Autodesk Inventor part; units mm, degrees
(part 2 of 2)
sketch "Sketch3" plane through (0, 0, -3.4) normal (0, 0, -1) x (-1, 0, 0)
  line L0 (0, 0) -> (23.6, 0)
  line L1 (23.6, 0) -> (23.6, 65.2958)
  line L2 (23.6, 65.2958) -> (0, 65.2958)
  line L3 (0, 65.2958) -> (0, 0)
  circle A0 centre (13, 35.0012) radius 9.6 construction
  circle A1 centre (8.9947, 46.9477) radius 8 construction
  circle A2 centre (8.9947, 46.9477) radius 8.4
  circle A3 centre (13, 35.0012) radius 10
  circle A4 centre (14.5, 55.2958) radius 5 projected
  circle A5 centre (8.9947, 46.9477) radius 1.25 construction
  arc A6 (9.7521, 54.9117) -> (9.2865, 53.8165) centre (14.0905, 52.4209) ccw construction
  arc A7 (9.2865, 53.8165) -> (8.9266, 53.8223) centre (8.9947, 46.9477) ccw construction
  arc A8 (8.9266, 53.8223) -> (8.4969, 54.9322) centre (4.0798, 52.5838) ccw construction
  arc A9 (8.4969, 54.9322) -> (8.0797, 54.8952) centre (8.9947, 46.9477) ccw construction
  arc A10 (8.0797, 54.8952) -> (7.852, 53.727) centre (12.8412, 53.3608) ccw construction
  arc A11 (7.852, 53.727) -> (7.4988, 53.6579) centre (8.9947, 46.9477) ccw construction
  arc A12 (7.4988, 53.6579) -> (6.8477, 54.6542) centre (3.0154, 51.4388) ccw construction
  arc A13 (6.8477, 54.6542) -> (6.4474, 54.5312) centre (8.9947, 46.9477) ccw construction
  arc A14 (6.4474, 54.5312) -> (6.4675, 53.3413) centre (11.4237, 54.0204) ccw construction
  arc A15 (6.4675, 53.3413) -> (6.1364, 53.2003) centre (8.9947, 46.9477) ccw construction
  arc A16 (6.1364, 53.2003) -> (5.2924, 54.0394) centre (2.2123, 50.0975) ccw construction
  arc A17 (5.2924, 54.0394) -> (4.9263, 53.8359) centre (8.9947, 46.9477) ccw construction
  arc A18 (4.9263, 53.8359) -> (5.1934, 52.6761) centre (9.9002, 54.3708) ccw construction
  arc A19 (5.1934, 52.6761) -> (4.8988, 52.4693) centre (8.9947, 46.9477) ccw construction
  arc A20 (4.8988, 52.4693) -> (3.8988, 53.1147) centre (1.7056, 48.6185) ccw construction
  arc A21 (3.8988, 53.1147) -> (3.5831, 52.8395) centre (8.9947, 46.9477) ccw construction
  arc A22 (3.5831, 52.8395) -> (4.0855, 51.7606) centre (8.337, 54.3968) ccw construction
  arc A23 (4.0855, 51.7606) -> (3.8403, 51.4971) centre (8.9947, 46.9477) ccw construction
  arc A24 (3.8403, 51.4971) -> (2.728, 51.9204) centre (1.5175, 47.0665) ccw construction
  arc A25 (2.728, 51.9204) -> (2.4763, 51.5856) centre (8.9947, 46.9477) ccw construction
  arc A26 (2.4763, 51.5856) -> (3.1921, 50.6348) centre (6.8026, 54.0973) ccw construction
  arc A27 (3.1921, 50.6348) -> (3.0071, 50.326) centre (8.9947, 46.9477) ccw construction
  arc A28 (3.0071, 50.326) -> (1.8311, 50.5088) centre (1.6562, 45.5093) ccw construction
  arc A29 (1.8311, 50.5088) -> (1.6545, 50.129) centre (8.9947, 46.9477) ccw construction
  arc A30 (1.6545, 50.129) -> (2.5523, 49.3477) centre (5.364, 53.4853) ccw construction
  arc A31 (2.5523, 49.3477) -> (2.4355, 49.0073) centre (8.9947, 46.9477) ccw construction
  arc A32 (2.4355, 49.0073) -> (1.2472, 48.9416) centre (2.1156, 44.015) ccw construction
  arc A33 (1.2472, 48.9416) -> (1.1535, 48.5334) centre (8.9947, 46.9477) ccw construction
  arc A34 (1.1535, 48.5334) -> (2.1941, 47.9558) centre (4.0841, 52.5876) ccw construction
  arc A35 (2.1941, 47.9558) -> (2.1506, 47.5985) centre (8.9947, 46.9477) ccw construction
  arc A36 (2.1506, 47.5985) -> (1.002, 47.2872) centre (2.8757, 42.6488) ccw construction
  arc A37 (1.002, 47.2872) -> (0.9951, 46.8684) centre (8.9947, 46.9477) ccw construction
  arc A38 (0.9951, 46.8684) -> (2.1331, 46.5199) centre (3.0188, 51.4434) ccw construction
  arc A39 (2.1331, 46.5199) -> (2.1649, 46.1613) centre (8.9947, 46.9477) ccw construction
  arc A40 (2.1649, 46.1613) -> (1.106, 45.618) centre (3.9032, 41.4705) ccw construction
  arc A41 (1.106, 45.618) -> (1.1864, 45.2069) centre (8.9947, 46.9477) ccw construction
  arc A42 (1.1864, 45.2069) -> (2.372, 45.1026) centre (2.2147, 50.1027) ccw construction
  arc A43 (2.372, 45.1026) -> (2.4776, 44.7585) centre (8.9947, 46.9477) ccw construction
  arc A44 (2.4776, 44.7585) -> (1.5549, 44.0069) centre (5.1532, 40.5316) ccw construction
  arc A45 (1.5549, 44.0069) -> (1.719, 43.6215) centre (8.9947, 46.9477) ccw construction
  arc A46 (1.719, 43.6215) -> (2.9003, 43.7659) centre (1.7069, 48.6241) ccw construction
  arc A47 (2.9003, 43.7659) -> (3.0752, 43.4513) centre (8.9947, 46.9477) ccw construction
  arc A48 (3.0752, 43.4513) -> (2.3289, 42.5243) centre (6.5711, 39.8731) ccw construction
  arc A49 (2.3289, 42.5243) -> (2.5695, 42.1815) centre (8.9947, 46.9477) ccw construction
  arc A50 (2.5695, 42.1815) -> (3.695, 42.5684) centre (1.5176, 47.0722) ccw construction
  arc A51 (3.695, 42.5684) -> (3.9314, 42.297) centre (8.9947, 46.9477) ccw construction
  arc A52 (3.9314, 42.297) -> (3.3942, 41.235) centre (8.095, 39.5238) ccw construction
  arc A53 (3.3942, 41.235) -> (3.7009, 40.9498) centre (8.9947, 46.9477) ccw construction
  arc A54 (3.7009, 40.9498) -> (4.7213, 41.5622) centre (1.6551, 45.5149) ccw construction
  arc A55 (4.7213, 41.5622) -> (5.009, 41.3459) centre (8.9947, 46.9477) ccw construction
  arc A56 (5.009, 41.3459) -> (4.7043, 40.1955) centre (9.6581, 39.499) ccw construction
  arc A57 (4.7043, 40.1955) -> (5.0636, 39.9802) centre (8.9947, 46.9477) ccw construction
  arc A58 (5.0636, 39.9802) -> (5.9344, 40.7914) centre (2.1134, 44.0202) ccw construction
  arc A59 (5.9344, 40.7914) -> (6.2608, 40.6396) centre (8.9947, 46.9477) ccw construction
  arc A60 (6.2608, 40.6396) -> (6.2019, 39.451) centre (11.1923, 39.7997) ccw construction
  arc A61 (6.2019, 39.451) -> (6.5981, 39.3151) centre (8.9947, 46.9477) ccw construction
  arc A62 (6.5981, 39.3151) -> (7.2812, 40.2896) centre (2.8724, 42.6535) ccw construction
  arc A63 (7.2812, 40.2896) -> (7.632, 40.2091) centre (8.9947, 46.9477) ccw construction
  arc A64 (7.632, 40.2091) -> (7.8216, 39.0341) centre (12.6304, 40.4128) ccw construction
  arc A65 (7.8216, 39.0341) -> (8.2374, 38.9836) centre (8.9947, 46.9477) ccw construction
  arc A66 (8.2374, 38.9836) -> (8.703, 40.0789) centre (3.899, 41.4744) ccw construction
  arc A67 (8.703, 40.0789) -> (9.0628, 40.073) centre (8.9947, 46.9477) ccw construction
  arc A68 (9.0628, 40.073) -> (9.4925, 38.9632) centre (13.9097, 41.3115) ccw construction
  arc A69 (9.4925, 38.9632) -> (9.9097, 39.0002) centre (8.9947, 46.9477) ccw construction
  arc A70 (9.9097, 39.0002) -> (10.1374, 40.1683) centre (5.1483, 40.5345) ccw construction
  arc A71 (10.1374, 40.1683) -> (10.4907, 40.2374) centre (8.9947, 46.9477) ccw construction
  arc A72 (10.4907, 40.2374) -> (11.1417, 39.2411) centre (14.9741, 42.4565) ccw construction
  arc A73 (11.1417, 39.2411) -> (11.5421, 39.3641) centre (8.9947, 46.9477) ccw construction
  arc A74 (11.5421, 39.3641) -> (11.522, 40.554) centre (6.5657, 39.875) ccw construction
  arc A75 (11.522, 40.554) -> (11.8531, 40.695) centre (8.9947, 46.9477) ccw construction
  arc A76 (11.8531, 40.695) -> (12.6971, 39.8559) centre (15.7772, 43.7978) ccw construction
  arc A77 (12.6971, 39.8559) -> (13.0632, 40.0594) centre (8.9947, 46.9477) ccw construction
  arc A78 (13.0632, 40.0594) -> (12.7961, 41.2192) centre (8.0893, 39.5245) ccw construction
  arc A79 (12.7961, 41.2192) -> (13.0907, 41.426) centre (8.9947, 46.9477) ccw construction
  arc A80 (13.0907, 41.426) -> (14.0906, 40.7807) centre (16.2839, 45.2768) ccw construction
  arc A81 (14.0906, 40.7807) -> (14.4064, 41.0558) centre (8.9947, 46.9477) ccw construction
  arc A82 (14.4064, 41.0558) -> (13.904, 42.1347) centre (9.6525, 39.4985) ccw construction
  arc A83 (13.904, 42.1347) -> (14.1492, 42.3982) centre (8.9947, 46.9477) ccw construction
  arc A84 (14.1492, 42.3982) -> (15.2615, 41.9749) centre (16.472, 46.8288) ccw construction
  arc A85 (15.2615, 41.9749) -> (15.5131, 42.3097) centre (8.9947, 46.9477) ccw construction
  arc A86 (15.5131, 42.3097) -> (14.7974, 43.2606) centre (11.1869, 39.798) ccw construction
  arc A87 (14.7974, 43.2606) -> (14.9824, 43.5693) centre (8.9947, 46.9477) ccw construction
  arc A88 (14.9824, 43.5693) -> (16.1584, 43.3865) centre (16.3333, 48.386) ccw construction
  arc A89 (16.1584, 43.3865) -> (16.335, 43.7663) centre (8.9947, 46.9477) ccw construction
  arc A90 (16.335, 43.7663) -> (15.4372, 44.5476) centre (12.6255, 40.41) ccw construction
  arc A91 (15.4372, 44.5476) -> (15.554, 44.888) centre (8.9947, 46.9477) ccw construction
  arc A92 (15.554, 44.888) -> (16.7423, 44.9538) centre (15.8739, 49.8803) ccw construction
  arc A93 (16.7423, 44.9538) -> (16.836, 45.362) centre (8.9947, 46.9477) ccw construction
  arc A94 (16.836, 45.362) -> (15.7954, 45.9395) centre (13.9054, 41.3077) ccw construction
  arc A95 (15.7954, 45.9395) -> (15.8389, 46.2968) centre (8.9947, 46.9477) ccw construction
  arc A96 (15.8389, 46.2968) -> (16.9875, 46.6081) centre (15.1138, 51.2465) ccw construction
  arc A97 (16.9875, 46.6081) -> (16.9944, 47.0269) centre (8.9947, 46.9477) ccw construction
  arc A98 (16.9944, 47.0269) -> (15.8564, 47.3755) centre (14.9707, 42.452) ccw construction
  arc A99 (15.8564, 47.3755) -> (15.8246, 47.734) centre (8.9947, 46.9477) ccw construction
  arc A100 (15.8246, 47.734) -> (16.8835, 48.2773) centre (14.0863, 52.4248) ccw construction
  arc A101 (16.8835, 48.2773) -> (16.8031, 48.6884) centre (8.9947, 46.9477) ccw construction
  arc A102 (16.8031, 48.6884) -> (15.6175, 48.7927) centre (15.7748, 43.7927) ccw construction
  arc A103 (15.6175, 48.7927) -> (15.5119, 49.1368) centre (8.9947, 46.9477) ccw construction
  arc A104 (15.5119, 49.1368) -> (16.4346, 49.8884) centre (12.8363, 53.3637) ccw construction
  arc A105 (16.4346, 49.8884) -> (16.2705, 50.2738) centre (8.9947, 46.9477) ccw construction
  arc A106 (16.2705, 50.2738) -> (15.0892, 50.1294) centre (16.2826, 45.2713) ccw construction
  arc A107 (15.0892, 50.1294) -> (14.9143, 50.444) centre (8.9947, 46.9477) ccw construction
  arc A108 (14.9143, 50.444) -> (15.6606, 51.371) centre (11.4184, 54.0222) ccw construction
  arc A109 (15.6606, 51.371) -> (15.42, 51.7138) centre (8.9947, 46.9477) ccw construction
  arc A110 (15.42, 51.7138) -> (14.2945, 51.3269) centre (16.4719, 46.8231) ccw construction
  arc A111 (14.2945, 51.3269) -> (14.058, 51.5983) centre (8.9947, 46.9477) ccw construction
  arc A112 (14.058, 51.5983) -> (14.5953, 52.6603) centre (9.8945, 54.3715) ccw construction
  arc A113 (14.5953, 52.6603) -> (14.2886, 52.9456) centre (8.9947, 46.9477) ccw construction
  arc A114 (14.2886, 52.9456) -> (13.2682, 52.3331) centre (16.3344, 48.3804) ccw construction
  arc A115 (13.2682, 52.3331) -> (12.9805, 52.5494) centre (8.9947, 46.9477) ccw construction
  arc A116 (12.9805, 52.5494) -> (13.2852, 53.6999) centre (8.3314, 54.3963) ccw construction
  arc A117 (13.2852, 53.6999) -> (12.9259, 53.9151) centre (8.9947, 46.9477) ccw construction
  arc A118 (12.9259, 53.9151) -> (12.0551, 53.1039) centre (15.8761, 49.8751) ccw construction
  arc A119 (12.0551, 53.1039) -> (11.7287, 53.2557) centre (8.9947, 46.9477) ccw construction
  arc A120 (11.7287, 53.2557) -> (11.7876, 54.4443) centre (6.7972, 54.0957) ccw construction
  arc A121 (11.7876, 54.4443) -> (11.3914, 54.5802) centre (8.9947, 46.9477) ccw construction
  arc A122 (11.3914, 54.5802) -> (10.7083, 53.6057) centre (15.1171, 51.2419) ccw construction
  arc A123 (10.7083, 53.6057) -> (10.3575, 53.6863) centre (8.9947, 46.9477) ccw construction
  arc A124 (10.3575, 53.6863) -> (10.1679, 54.8612) centre (5.3591, 53.4826) ccw construction
  arc A125 (10.1679, 54.8612) -> (9.7521, 54.9117) centre (8.9947, 46.9477) ccw construction
  arc A126 (6.571, 40.1714) -> (5.2144, 40.6176) centre (4.0302, 34.7325) ccw construction
  arc A127 (5.2144, 40.6176) -> (4.9311, 40.2025) centre (13, 35.0012) ccw construction
  arc A128 (4.9311, 40.2025) -> (5.8414, 39.102) centre (9.9791, 43.4512) ccw construction
  arc A129 (5.8414, 39.102) -> (5.6366, 38.7217) centre (13, 35.0012) ccw construction
  arc A130 (5.6366, 38.7217) -> (4.2168, 38.8762) centre (4.2821, 32.8735) ccw construction
  arc A131 (4.2168, 38.8762) -> (4.026, 38.4112) centre (13, 35.0012) ccw construction
  arc A132 (4.026, 38.4112) -> (5.1452, 37.524) centre (8.2882, 42.6385) ccw construction
  arc A133 (5.1452, 37.524) -> (5.0239, 37.1095) centre (13, 35.0012) ccw construction
  arc A134 (5.0239, 37.1095) -> (3.6031, 36.9654) centre (4.915, 31.1074) ccw construction
  arc A135 (3.6031, 36.9654) -> (3.5132, 36.4709) centre (13, 35.0012) ccw construction
  arc A136 (3.5132, 36.4709) -> (4.7923, 35.8358) centre (6.8033, 41.492) ccw construction
  arc A137 (4.7923, 35.8358) -> (4.7599, 35.4051) centre (13, 35.0012) ccw construction
  arc A138 (4.7599, 35.4051) -> (3.4001, 34.9687) centre (5.9012, 29.5115) ccw construction
  arc A139 (3.4001, 34.9687) -> (3.4149, 34.4663) centre (13, 35.0012) ccw construction
  arc A140 (3.4149, 34.4663) -> (4.7982, 34.1111) centre (5.5892, 40.0618) ccw construction
  arc A141 (4.7982, 34.1111) -> (4.856, 33.6831) centre (13, 35.0012) ccw construction
  arc A142 (4.856, 33.6831) -> (3.6166, 32.9735) centre (7.1977, 28.1556) ccw construction
  arc A143 (3.6166, 32.9735) -> (3.7356, 32.4852) centre (13, 35.0012) ccw construction
  arc A144 (3.7356, 32.4852) -> (5.1625, 32.4253) centre (4.699, 38.4104) ccw construction
  arc A145 (5.1625, 32.4253) -> (5.308, 32.0186) centre (13, 35.0012) ccw construction
  arc A146 (5.308, 32.0186) -> (4.2432, 31.0669) centre (8.7478, 27.0988) ccw construction
  arc A147 (4.2432, 31.0669) -> (4.4611, 30.614) centre (13, 35.0012) ccw construction
  arc A148 (4.4611, 30.614) -> (5.8693, 30.8521) centre (4.1716, 36.61) ccw construction
  arc A149 (5.8693, 30.8521) -> (6.0962, 30.4845) centre (13, 35.0012) ccw construction
  arc A150 (6.0962, 30.4845) -> (5.2526, 29.3322) centre (10.4837, 26.3874) ccw construction
  arc A151 (5.2526, 29.3322) -> (5.5599, 28.9345) centre (13, 35.0012) ccw construction
  arc A152 (5.5599, 28.9345) -> (6.8878, 29.4602) centre (4.03, 34.7394) ccw construction
  arc A153 (6.8878, 29.4602) -> (7.1861, 29.1479) centre (13, 35.0012) ccw construction
  arc A154 (7.1861, 29.1479) -> (6.6005, 27.8453) centre (12.3296, 26.0525) ccw construction
  arc A155 (6.6005, 27.8453) -> (6.9838, 27.5202) centre (13, 35.0012) ccw construction
  arc A156 (6.9838, 27.5202) -> (8.1734, 28.3104) centre (4.2805, 32.8801) ccw construction
  arc A157 (8.1734, 28.3104) -> (8.5302, 28.067) centre (13, 35.0012) ccw construction
  arc A158 (8.5302, 28.067) -> (8.2282, 26.6712) centre (14.2048, 26.1086) ccw construction
  arc A159 (8.2282, 26.6712) -> (8.6707, 26.4328) centre (13, 35.0012) ccw construction
  arc A160 (8.6707, 26.4328) -> (9.6699, 27.4531) centre (4.912, 31.1136) ccw construction
  arc A161 (9.6699, 27.4531) -> (10.0695, 27.2892) centre (13, 35.0012) ccw construction
  arc A162 (10.0695, 27.2892) -> (10.0643, 25.8611) centre (16.0273, 26.5534) ccw construction
  arc A163 (10.0643, 25.8611) -> (10.5467, 25.72) centre (13, 35.0012) ccw construction
  arc A164 (10.5467, 25.72) -> (11.312, 26.9257) centre (5.897, 29.5169) ccw construction
  arc A165 (11.312, 26.9257) -> (11.737, 26.8485) centre (13, 35.0012) ccw construction
  arc A166 (11.737, 26.8485) -> (12.0288, 25.4504) centre (17.7176, 27.3675) ccw construction
  arc A167 (12.0288, 25.4504) -> (12.53, 25.4127) centre (13, 35.0012) ccw construction
  arc A168 (12.53, 25.4127) -> (13.0279, 26.7512) centre (7.1925, 28.16) ccw construction
  arc A169 (13.0279, 26.7512) -> (13.4596, 26.764) centre (13, 35.0012) ccw construction
  arc A170 (13.4596, 26.764) -> (14.0358, 25.4572) centre (19.2016, 28.5151) ccw construction
  arc A171 (14.0358, 25.4572) -> (14.5338, 25.5245) centre (13, 35.0012) ccw construction
  arc A172 (14.5338, 25.5245) -> (14.7426, 26.9373) centre (8.7418, 27.102) ccw construction
  arc A173 (14.7426, 26.9373) -> (15.1622, 27.0396) centre (13, 35.0012) ccw construction
  arc A174 (15.1622, 27.0396) -> (15.9974, 25.8811) centre (20.4146, 29.9462) ccw construction
  arc A175 (15.9974, 25.8811) -> (16.4706, 26.0505) centre (13, 35.0012) ccw construction
  arc A176 (16.4706, 26.0505) -> (16.3811, 27.4758) centre (10.4772, 26.3893) ccw construction
  arc A177 (16.3811, 27.4758) -> (16.7703, 27.6631) centre (13, 35.0012) ccw construction
  arc A178 (16.7703, 27.6631) -> (17.8281, 26.7036) centre (21.3036, 31.5983) ccw construction
  arc A179 (17.8281, 26.7036) -> (18.2557, 26.9677) centre (13, 35.0012) ccw construction
  arc A180 (18.2557, 26.9677) -> (17.8718, 28.3432) centre (12.3228, 26.053) ccw construction
  arc A181 (17.8718, 28.3432) -> (18.2136, 28.6073) centre (13, 35.0012) ccw construction
  arc A182 (18.2136, 28.6073) -> (19.4477, 27.8888) centre (21.8296, 33.3991) ccw construction
  arc A183 (19.4477, 27.8888) -> (19.8111, 28.236) centre (13, 35.0012) ccw construction
  arc A184 (19.8111, 28.236) -> (19.1496, 29.5016) centre (14.198, 26.1077) ccw construction
  arc A185 (19.1496, 29.5016) -> (19.429, 29.831) centre (13, 35.0012) ccw construction
  arc A186 (19.429, 29.831) -> (20.7856, 29.3848) centre (21.9698, 35.2699) ccw construction
  arc A187 (20.7856, 29.3848) -> (21.0689, 29.7999) centre (13, 35.0012) ccw construction
  arc A188 (21.0689, 29.7999) -> (20.1586, 30.9004) centre (16.0209, 26.5512) ccw construction
  arc A189 (20.1586, 30.9004) -> (20.3634, 31.2807) centre (13, 35.0012) ccw construction
  arc A190 (20.3634, 31.2807) -> (21.7832, 31.1262) centre (21.7179, 37.1289) ccw construction
  arc A191 (21.7832, 31.1262) -> (21.974, 31.5912) centre (13, 35.0012) ccw construction
  arc A192 (21.974, 31.5912) -> (20.8548, 32.4784) centre (17.7118, 27.3639) ccw construction
  arc A193 (20.8548, 32.4784) -> (20.9761, 32.8929) centre (13, 35.0012) ccw construction
  arc A194 (20.9761, 32.8929) -> (22.3969, 33.037) centre (21.085, 38.895) ccw construction
  arc A195 (22.3969, 33.037) -> (22.4868, 33.5315) centre (13, 35.0012) ccw construction
  arc A196 (22.4868, 33.5315) -> (21.2077, 34.1666) centre (19.1967, 28.5104) ccw construction
  arc A197 (21.2077, 34.1666) -> (21.2401, 34.5973) centre (13, 35.0012) ccw construction
  arc A198 (21.2401, 34.5973) -> (22.5999, 35.0337) centre (20.0988, 40.4909) ccw construction
  arc A199 (22.5999, 35.0337) -> (22.5851, 35.5361) centre (13, 35.0012) ccw construction
  arc A200 (22.5851, 35.5361) -> (21.2018, 35.8913) centre (20.4108, 29.9406) ccw construction
  arc A201 (21.2018, 35.8913) -> (21.144, 36.3193) centre (13, 35.0012) ccw construction
  arc A202 (21.144, 36.3193) -> (22.3834, 37.0289) centre (18.8023, 41.8468) ccw construction
  arc A203 (22.3834, 37.0289) -> (22.2644, 37.5172) centre (13, 35.0012) ccw construction
  arc A204 (22.2644, 37.5172) -> (20.8375, 37.5771) centre (21.301, 31.592) ccw construction
  arc A205 (20.8375, 37.5771) -> (20.692, 37.9838) centre (13, 35.0012) ccw construction
  arc A206 (20.692, 37.9838) -> (21.7568, 38.9355) centre (17.2522, 42.9036) ccw construction
  arc A207 (21.7568, 38.9355) -> (21.5389, 39.3884) centre (13, 35.0012) ccw construction
  arc A208 (21.5389, 39.3884) -> (20.1307, 39.1503) centre (21.8284, 33.3924) ccw construction
  arc A209 (20.1307, 39.1503) -> (19.9038, 39.5178) centre (13, 35.0012) ccw construction
  arc A210 (19.9038, 39.5178) -> (20.7474, 40.6702) centre (15.5163, 43.615) ccw construction
  arc A211 (20.7474, 40.6702) -> (20.4401, 41.0679) centre (13, 35.0012) ccw construction
  arc A212 (20.4401, 41.0679) -> (19.1122, 40.5422) centre (21.97, 35.263) ccw construction
  arc A213 (19.1122, 40.5422) -> (18.8139, 40.8545) centre (13, 35.0012) ccw construction
  arc A214 (18.8139, 40.8545) -> (19.3995, 42.1571) centre (13.6704, 43.9499) ccw construction
  arc A215 (19.3995, 42.1571) -> (19.0162, 42.4822) centre (13, 35.0012) ccw construction
  arc A216 (19.0162, 42.4822) -> (17.8266, 41.692) centre (21.7195, 37.1223) ccw construction
  arc A217 (17.8266, 41.692) -> (17.4698, 41.9354) centre (13, 35.0012) ccw construction
  arc A218 (17.4698, 41.9354) -> (17.7718, 43.3312) centre (11.7952, 43.8938) ccw construction
  arc A219 (17.7718, 43.3312) -> (17.3293, 43.5696) centre (13, 35.0012) ccw construction
  arc A220 (17.3293, 43.5696) -> (16.3301, 42.5493) centre (21.088, 38.8888) ccw construction
  arc A221 (16.3301, 42.5493) -> (15.9305, 42.7132) centre (13, 35.0012) ccw construction
  arc A222 (15.9305, 42.7132) -> (15.9357, 44.1413) centre (9.9727, 43.4489) ccw construction
  arc A223 (15.9357, 44.1413) -> (15.4533, 44.2824) centre (13, 35.0012) ccw construction
  arc A224 (15.4533, 44.2824) -> (14.688, 43.0767) centre (20.103, 40.4855) ccw construction
  arc A225 (14.688, 43.0767) -> (14.263, 43.1539) centre (13, 35.0012) ccw construction
  arc A226 (14.263, 43.1539) -> (13.9712, 44.5519) centre (8.2824, 42.6349) ccw construction
  arc A227 (13.9712, 44.5519) -> (13.47, 44.5897) centre (13, 35.0012) ccw construction
  arc A228 (13.47, 44.5897) -> (12.9721, 43.2512) centre (18.8075, 41.8424) ccw construction
  arc A229 (12.9721, 43.2512) -> (12.5404, 43.2384) centre (13, 35.0012) ccw construction
  arc A230 (12.5404, 43.2384) -> (11.9642, 44.5452) centre (6.7984, 41.4873) ccw construction
  arc A231 (11.9642, 44.5452) -> (11.4662, 44.4779) centre (13, 35.0012) ccw construction
  arc A232 (11.4662, 44.4779) -> (11.2574, 43.0651) centre (17.2582, 42.9004) ccw construction
  arc A233 (11.2574, 43.0651) -> (10.8378, 42.9628) centre (13, 35.0012) ccw construction
  arc A234 (10.8378, 42.9628) -> (10.0026, 44.1213) centre (5.5854, 40.0562) ccw construction
  arc A235 (10.0026, 44.1213) -> (9.5294, 43.9519) centre (13, 35.0012) ccw construction
  arc A236 (9.5294, 43.9519) -> (9.6189, 42.5266) centre (15.5228, 43.6131) ccw construction
  arc A237 (9.6189, 42.5266) -> (9.2297, 42.3393) centre (13, 35.0012) ccw construction
  arc A238 (9.2297, 42.3393) -> (8.1719, 43.2988) centre (4.6964, 38.4041) ccw construction
  arc A239 (8.1719, 43.2988) -> (7.7443, 43.0347) centre (13, 35.0012) ccw construction
  arc A240 (7.7443, 43.0347) -> (8.1282, 41.6591) centre (13.6772, 43.9494) ccw construction
  arc A241 (8.1282, 41.6591) -> (7.7864, 41.3951) centre (13, 35.0012) ccw construction
  arc A242 (7.7864, 41.3951) -> (6.5523, 42.1136) centre (4.1704, 36.6033) ccw construction
  arc A243 (6.5523, 42.1136) -> (6.1889, 41.7664) centre (13, 35.0012) ccw construction
  arc A244 (6.1889, 41.7664) -> (6.8504, 40.5008) centre (11.802, 43.8947) ccw construction
  arc A245 (6.8504, 40.5008) -> (6.571, 40.1714) centre (13, 35.0012) ccw construction
  point P0 (16.2655, 43.6106)
  point P1 (4.3207, 39.9681)
  point P2 (16.9313, 44.196)
  point P3 (16.846, 48.4834)
  point P4 (16.5028, 50.7145)
  point P5 (9.5001, 55.3324)
  dimension "d21" = 0.4
  dimension "d22" = 0.4
  constraints: 8 end point, 3 centre point, 3 point on circle, 2 coincident, 2 parallel, 1 horizontal, 1 perpendicular, 3 other
  measures "d21" radial gap between concentric circles of A1 A2
extrude "Extrusion7" add sketch "Sketch3" along normal blind 3.7
sketch "Sketch12" plane through (-34.0123, 35.7835, 2.1) normal (0, 0, -1) x (-0.6427876, 0.7660444, 0)
  circle A0 centre (-7.5288, 26.3408) radius 1.25 construction
  arc A1 (-9.9487, 22.908) -> (-8.8528, 23.817) centre (-11.7217, 26.1608) ccw construction
  arc A2 (-8.8528, 23.817) -> (-8.512, 23.6657) centre (-7.5288, 26.3408) ccw construction
  arc A3 (-8.512, 23.6657) -> (-8.4509, 22.2432) centre (-4.8493, 23.1107) ccw construction
  arc A4 (-8.4509, 22.2432) -> (-7.9081, 22.1579) centre (-7.5288, 26.3408) ccw construction
  arc A5 (-7.9081, 22.1579) -> (-7.4135, 23.4931) centre (-11.0699, 24.0884) ccw construction
  arc A6 (-7.4135, 23.4931) -> (-7.0428, 23.5325) centre (-7.5288, 26.3408) ccw construction
  arc A7 (-7.0428, 23.5325) -> (-6.2786, 22.3311) centre (-3.5933, 24.8832) ccw construction
  arc A8 (-6.2786, 22.3311) -> (-5.7659, 22.5286) centre (-7.5288, 26.3408) ccw construction
  arc A9 (-5.7659, 22.5286) -> (-6.0051, 23.9322) centre (-9.4693, 22.6196) ccw construction
  arc A10 (-6.0051, 23.9322) -> (-5.7038, 24.1517) centre (-7.5288, 26.3408) ccw construction
  arc A11 (-5.7038, 24.1517) -> (-4.4412, 23.4934) centre (-3.3917, 27.0462) ccw construction
  arc A12 (-4.4412, 23.4934) -> (-4.096, 23.9208) centre (-7.5288, 26.3408) ccw construction
  arc A13 (-4.096, 23.9208) -> (-5.005, 25.0167) centre (-7.3488, 22.1479) ccw construction
  arc A14 (-5.005, 25.0167) -> (-4.8538, 25.3575) centre (-7.5288, 26.3408) ccw construction
  arc A15 (-4.8538, 25.3575) -> (-3.4312, 25.4187) centre (-4.2987, 29.0202) ccw construction
  arc A16 (-3.4312, 25.4187) -> (-3.3459, 25.9614) centre (-7.5288, 26.3408) ccw construction
  arc A17 (-3.3459, 25.9614) -> (-4.6811, 26.456) centre (-5.2764, 22.7996) ccw construction
  arc A18 (-4.6811, 26.456) -> (-4.7205, 26.8267) centre (-7.5288, 26.3408) ccw construction
  arc A19 (-4.7205, 26.8267) -> (-3.5192, 27.591) centre (-6.0712, 30.2763) ccw construction
  arc A20 (-3.5192, 27.591) -> (-3.7166, 28.1036) centre (-7.5288, 26.3408) ccw construction
  arc A21 (-3.7166, 28.1036) -> (-5.1202, 27.8644) centre (-3.8076, 24.4002) ccw construction
  arc A22 (-5.1202, 27.8644) -> (-5.3397, 28.1657) centre (-7.5288, 26.3408) ccw construction
  arc A23 (-5.3397, 28.1657) -> (-4.6814, 29.4283) centre (-8.2342, 30.4778) ccw construction
  arc A24 (-4.6814, 29.4283) -> (-5.1088, 29.7735) centre (-7.5288, 26.3408) ccw construction
  arc A25 (-5.1088, 29.7735) -> (-6.2047, 28.8645) centre (-3.3359, 26.5207) ccw construction
  arc A26 (-6.2047, 28.8645) -> (-6.5455, 29.0158) centre (-7.5288, 26.3408) ccw construction
  arc A27 (-6.5455, 29.0158) -> (-6.6067, 30.4383) centre (-10.2082, 29.5708) ccw construction
  arc A28 (-6.6067, 30.4383) -> (-7.1494, 30.5236) centre (-7.5288, 26.3408) ccw construction
  arc A29 (-7.1494, 30.5236) -> (-7.644, 29.1884) centre (-3.9876, 28.5931) ccw construction
  arc A30 (-7.644, 29.1884) -> (-8.0147, 29.149) centre (-7.5288, 26.3408) ccw construction
  arc A31 (-8.0147, 29.149) -> (-8.779, 30.3504) centre (-11.4643, 27.7983) ccw construction
  arc A32 (-8.779, 30.3504) -> (-9.2916, 30.1529) centre (-7.5288, 26.3408) ccw construction
  arc A33 (-9.2916, 30.1529) -> (-9.0524, 28.7493) centre (-5.5882, 30.0619) ccw construction
  arc A34 (-9.0524, 28.7493) -> (-9.3537, 28.5298) centre (-7.5288, 26.3408) ccw construction
  arc A35 (-9.3537, 28.5298) -> (-10.6163, 29.1881) centre (-11.6658, 25.6353) ccw construction
  arc A36 (-10.6163, 29.1881) -> (-10.9615, 28.7607) centre (-7.5288, 26.3408) ccw construction
  arc A37 (-10.9615, 28.7607) -> (-10.0525, 27.6648) centre (-7.7088, 30.5336) ccw construction
  arc A38 (-10.0525, 27.6648) -> (-10.2038, 27.324) centre (-7.5288, 26.3408) ccw construction
  arc A39 (-10.2038, 27.324) -> (-11.6263, 27.2628) centre (-10.7588, 23.6613) ccw construction
  arc A40 (-11.6263, 27.2628) -> (-11.7116, 26.7201) centre (-7.5288, 26.3408) ccw construction
  arc A41 (-11.7116, 26.7201) -> (-10.3764, 26.2255) centre (-9.7811, 29.8819) ccw construction
  arc A42 (-10.3764, 26.2255) -> (-10.337, 25.8548) centre (-7.5288, 26.3408) ccw construction
  arc A43 (-10.337, 25.8548) -> (-11.5384, 25.0905) centre (-8.9863, 22.4052) ccw construction
  arc A44 (-11.5384, 25.0905) -> (-11.3409, 24.5779) centre (-7.5288, 26.3408) ccw construction
  arc A45 (-11.3409, 24.5779) -> (-9.9373, 24.8171) centre (-11.2499, 28.2813) ccw construction
  arc A46 (-9.9373, 24.8171) -> (-9.7178, 24.5158) centre (-7.5288, 26.3408) ccw construction
  arc A47 (-9.7178, 24.5158) -> (-10.3761, 23.2532) centre (-6.8233, 22.2037) ccw construction
  arc A48 (-10.3761, 23.2532) -> (-9.9487, 22.908) centre (-7.5288, 26.3408) ccw construction
  circle A49 centre (-7.5288, 26.3408) radius 4.2 construction
  circle A50 centre (-7.5288, 26.3408) radius 4.6
  point P0 (-49.2745, 3.0538)
  dimension "d128" = 0.4
  constraints: 1 centre point, 1 coincident, 3 other
extrude "Extrusion11" add sketch "Sketch12" along normal blind 1.5
ref_plane "Work Plane8" through (-34.0123, -5.0123, 0) normal (0, 0, -1) x (0.6427876, 0.7660444, 0)
sketch "Sketch4" plane through (0, 0, -7.1) normal (0, 0, -1) x (-1, 0, 0)
  line L0 (1.5, 0.5) -> (1.5, 16.5) projected
  line L1 (2.5, 0.5) -> (1.5, 0.5) projected
  line L2 (2.5, 16.5) -> (2.5, 0.5) projected
  line L3 (2.5, 16.5) -> (1.5, 16.5) projected
  line L4 (2.5, 16.5) -> (2.5, 17)
  line L5 (2.5, 17) -> (1, 17)
  line L6 (1, 17) -> (1, 0.5)
  line L7 (23.6, 0) -> (0, 0) projected
  line L8 (1, 0.5) -> (1.5, 0.5)
  dimension "d27" = 0.5
  dimension "d28" = 0.5
  constraints: 8 end point, 2 perpendicular, 1 collinear, 1 vertical
  measures "d27" distance between parallel lines of L5 L3
  measures "d28" distance between parallel lines of L6 L0
extrude "Extrusion8" cut sketch "Sketch4" against normal blind 7.1
sketch "Sketch9" plane through (0, 0, 0.6) normal (0, 0, -1) x (-1, 0, 0)
  arc A0 (9.5001, 55.3324) -> (4.3207, 39.9681) centre (8.9947, 46.9477) ccw projected
  point P0 (0, 0)
  point P1 (16.9313, 44.196)
hole "Hole3" at (-8.9947, 46.9477, 0.6) direction (0, 0, 1) diameter 2.5 depth 1.3
sketch "Sketch5" plane through (0, 0, -7.1) normal (0, 0, -1) x (-1, 0, 0)
  line L0 (1.5, 0.5) -> (1.5, 16.5) projected
  line L1 (2.5, 0.5) -> (1.5, 0.5) projected
  line L2 (2.5, 16.5) -> (2.5, 0.5) projected
  line L3 (2.5, 16.5) -> (1.5, 16.5) projected
  line L4 (2.5, 16.5) -> (2.5, 18)
  line L5 (2.5, 18) -> (0, 18)
  line L6 (0, 0) -> (0, 65.2958) projected
  line L7 (0, 0) -> (0, 18)
  line L8 (0, 0) -> (2.5, 0)
  line L9 (2.5, 0) -> (2.5, 0.5)
  line L10 (1, 17) -> (1, 0)
  line L11 (1, 0) -> (3, 0)
  line L12 (3, 0) -> (3, 17)
  line L13 (3, 17) -> (1, 17)
  line L14 (1.5, 13.4) -> (1.5, 9.9) projected
  line L15 (1.5, 13.4) -> (0, 13.4) projected
  line L16 (0, 9.9) -> (0, 13.4) projected
  line L17 (1.5, 9.9) -> (0, 9.9) projected
  line L18 (1.5, 7.1) -> (1.5, 3.6) projected
  line L19 (1.5, 7.1) -> (0, 7.1) projected
  line L20 (0, 3.6) -> (0, 7.1) projected
  line L21 (1.5, 3.6) -> (0, 3.6) projected
  line L22 (-0.5, 13.9) -> (2, 13.9)
  line L23 (2, 13.9) -> (2, 9.4)
  line L24 (2, 9.4) -> (-0.5, 9.4)
  line L25 (-0.5, 9.4) -> (-0.5, 13.9)
  line L26 (-0.5, 7.6) -> (2, 7.6)
  line L27 (2, 7.6) -> (2, 3.1)
  line L28 (2, 3.1) -> (-0.5, 3.1)
  line L29 (-0.5, 3.1) -> (-0.5, 7.6)
  line L30 (1.5, 0.5) -> (1, 0.5)
  point P0 (0, 13.9)
  point P1 (1, 13.9)
  point P2 (2.5, 17)
  point P3 (0, 7.6)
  point P4 (1, 7.6)
  point P5 (1, 9.4)
  point P6 (0, 9.4)
  point P7 (1, 3.1)
  point P8 (0, 3.1)
  point P9 (0, 3.1)
  point P10 (0, 7.6)
  point P11 (2.5, 0)
  point P12 (1, 0)
  dimension "d31" = 0.5
  dimension "d32" = 1
  dimension "d33" = 0.5
  dimension "d34" = 0.5
  constraints: 36 end point, 3 perpendicular, 3 point on line, 2 collinear, 1 vertical, 9 other
  measures "d31" distance between parallel lines of L0 L10
  measures "d32" distance between parallel lines of L5 L13
  measures "d33" distance between parallel lines of L15 L22
  measures "d34" distance between parallel lines of L19 L26
ref_plane "Work Plane6" through (-2.5, 0.5, -17) normal (0, 0, -1) x (0, 1, 0)
extrude "Extrusion9" add sketch "Sketch5" along normal blind 8 contours L1 L9 L8 L10 L30 | L10 L8 L6 L28 | L13 L10 L22 L6 L5 L4
sketch "Sketch7" plane through (0, 0, -7.1) normal (0, 0, -1) x (-1, 0, 0)
  circle A0 centre (8.3716, 60.4381) radius 1.0564 projected
  circle A1 centre (20.6284, 50.1535) radius 1.0564 projected
  circle A2 centre (14.5, 55.2958) radius 5 projected
  circle A3 centre (14.5, 55.2958) radius 13.85 projected
  circle A4 centre (8.3716, 60.4381) radius 2.25
  circle A5 centre (20.6284, 50.1535) radius 2.25
  point P0 (0, 0)
  dimension "d132" = 4.5
  dimension "d133" = 4.5
  constraints: 2 centre point, 2 coincident
  measures "d132" diameter of A4
  measures "d133" diameter of A5
extrude "Extrusion10" cut sketch "Sketch7" against normal blind 2.7 contours A0 | A1 | A4 | A5
sketch "Sketch8" plane through (-8.3716, 63.2121, -4.4) normal (0, 0, -1) x (-1, 0, 0)
  circle A0 centre (0, -2.774) radius 1.0564 projected
  circle A1 centre (12.2567, -13.0586) radius 1.0564 projected
  circle A2 centre (6.1284, -7.9163) radius 5 projected
  circle A3 centre (6.1284, -7.9163) radius 13.85 projected
  point P0 (-8.3716, -63.2121)
  point P1 (0, 0)
  point P2 (12.2567, -10.2846)
hole "Hole2" at (-20.6284, 50.1535, -4.4) at (-8.3716, 60.4381, -4.4) direction (0, 0, 1) diameter 2.5 depth 8.8 counterbore diameter 4.5 counterbore depth 2.5
sketch "Sketch6" plane through (-23.6, 65.2958, 2.1) normal (0, 1, 0) x (1, 0, 0)
  line L0 (0, 9.2) -> (0, 0) projected
  line L1 (23.6, 0) -> (0, 0) projected
  line L2 (0, 4.6) -> (23.6, 4.6)
  line L3 (0.6, 9.2) -> (20.6, 9.2) projected
  line L4 (17.6, 9.2) -> (17.6, 0)
  circle A0 centre (11.1, 4.6) radius 3.5
  circle A1 centre (3.5, 4.6) radius 3.5
  line L5 (23.6, 9.2) -> (23.6, 0) projected
  line L6 (0, 9.2) -> (23.6, 9.2) projected
  point P0 (23.6, 2.1)
  point P1 (11.8, 4.6)
  point P2 (19.8, 4.6)
  point P3 (19.2793, 9.2)
  point P4 (6.6687, 9.2)
  dimension "d52" = 7
  dimension "d53" = 7
  dimension "d55" = 0
  dimension "d67" = 3
  dimension "d102" = 6
  constraints: 5 point on line, 4 end point, 3 midpoint, 2 centre point, 1 perpendicular
  measures "d52" diameter of A1
  measures "d53" diameter of A0
  measures "d55" distance edge to line of A1 L0
  measures "d67" distance edge to line of A0 L4
  measures "d102" distance between parallel lines of L5 L4
hole "Hole1" at (-20.1, 65.2958, -2.5) at (-12.5, 65.2958, -2.5) direction (0, -1, 0) diameter 4 depth 4 counterbore diameter 4.5 counterbore depth 0.5
sketch "Sketch10" plane through (0, 0, -7.1) normal (0, 0, -1) x (-1, 0, 0)
  line L0 (23.6, 0) -> (23.6, 65.2958) projected
  line L1 (23.6, 4.75) -> (0, 4.75)
  line L2 (0, 0) -> (0, 65.2958) projected
  line L3 (0, 13) -> (23.6, 13)
  line L4 (23.6, 19) -> (0, 19)
  circle A0 centre (3.5, 61.7958) radius 3.5
  circle A1 centre (3.5, 61.7958) radius 2.5
  line L5 (23.6, 65.2958) -> (0, 65.2958) projected
  line L6 (0, 65.2958) -> (0, 0) projected
  circle A2 centre (19.8282, 45.4714) radius 3.5
  circle A3 centre (19.8282, 45.4714) radius 2.5
  circle A4 centre (3.5, 25.4095) radius 3.5
  circle A5 centre (20.1, 22.5) radius 3.5
  line L7 (23.6, 0) -> (23.6, 65.2958) projected
  circle A6 centre (7, 8.875) radius 3.5
  circle A7 centre (19.6, 8.875) radius 3.5
  line L8 (2.5, 0) -> (23.6, 0) projected
  line L9 (23.6, 65.2958) -> (0, 65.2958) projected
  line L10 (0, 18) -> (2.5, 18) projected
  line L11 (2.5, 18) -> (2.5, 17) projected
  line L12 (1, 13.9) -> (0, 13.9) projected
  line L13 (0, 13.9) -> (0, 3.1) projected
  line L14 (1, 3.1) -> (1, 13.9) projected
  line L15 (0, 65.2958) -> (0, 18) projected
  circle A8 centre (8.3716, 60.4381) radius 2.25 projected
  circle A9 centre (20.6284, 50.1535) radius 2.25 projected
  line L16 (2.5, 0) -> (23.6, 0) projected
  line L17 (23.6, 0) -> (23.6, 65.2958) projected
  line L18 (23.6, 65.2958) -> (0, 65.2958) projected
  line L19 (0, 65.2958) -> (0, 18) projected
  line L20 (0, 18) -> (2.5, 18) projected
  line L21 (2.5, 18) -> (2.5, 17) projected
  arc A10 (16.5028, 50.7145) -> (9.5001, 55.3324) centre (14.5, 55.2958) ccw projected
  arc A11 (16.9313, 44.196) -> (16.5028, 50.7145) centre (8.9947, 46.9477) ccw projected
  arc A12 (4.3207, 39.9681) -> (16.9313, 44.196) centre (13, 35.0012) ccw projected
  arc A13 (9.5001, 55.3324) -> (4.3207, 39.9681) centre (8.9947, 46.9477) ccw projected
  arc A14 (4.3207, 39.9681) -> (16.9313, 44.196) centre (13, 35.0012) ccw projected
  line L22 (2.5, 17) -> (2.5, 0.5) projected
  line L23 (2.5, 0.5) -> (2.5, 0) projected
  line L24 (2.5, 17) -> (2.5, 0.5) projected
  line L25 (2.5, 0.5) -> (2.5, 0) projected
  line L26 (0, 3.1) -> (1, 3.1) projected
  point P0 (23.2, 52.8075)
  point P1 (23.2, 54.1548)
  point P2 (23.2, -23.4755)
  point P3 (23.2, -18.5366)
  dimension "d77" = 8.25
  dimension "d78" = 6
  dimension "d79" = 7
  dimension "d80" = 5
  dimension "d81" = 7
  dimension "d82" = 5
  dimension "d86" = 7
  dimension "d87" = 7
  dimension "d88" = 7
  dimension "d89" = 7
  dimension "d90" = 4.125
  dimension "d91" = 4.125
  dimension "d92" = 7
  dimension "d93" = 4
  dimension "d94" = 4.125
  constraints: 8 centre point, 7 tangent, 6 end point, 6 point on line, 2 coincident, 1 horizontal, 1 perpendicular, 2 other
  measures "d77" distance between parallel lines of L3 L1
  measures "d78" distance between parallel lines of L3 L4
  measures "d79" diameter of A0
  measures "d80" diameter of A1
  measures "d81" diameter of A2
  measures "d82" diameter of A3
  measures "d86" diameter of A4
  measures "d87" diameter of A5
  measures "d88" diameter of A6
  measures "d89" distance from line of L2 A6.centre
  measures "d90" distance from line of L3 A6.centre
  measures "d91" distance from line of L1 A6.centre
  measures "d92" diameter of A7
  measures "d94" distance from line of L3 A7.centre
hole "Hole4" at (-3.5, 61.7958, -7.1) at (-19.8282, 45.4714, -7.1) at (-20.1, 22.5, -7.1) at (-3.5, 25.4095, -7.1) at (-7, 8.875, -7.1) at (-19.6, 8.875, -7.1) direction (0, 0, 1) diameter 4 depth 3.5 counterbore diameter 4.5 counterbore depth 0.5
sketch "Sketch11" plane through (-23.6, 24.9409, 2.1) normal (-1, 0, 0) x (0, 0, 1)
  circle A0 centre (-6.6928, -22.4337) radius 2.5072
  line L0 (-9.2, -24.9409) -> (-9.2, 40.3549) projected
  line L1 (-2.1, -24.9409) -> (0, -24.9409) projected
  line L2 (-2.1, -5.4409) -> (-2.1, -15.4409) projected
  line L3 (-2.1, -16.2127) -> (-3.1, -16.2127) projected
  line L4 (-2.1, -6.0686) -> (-2.1, -16.2127) projected
  line L5 (-2.1, -12.0127) -> (-9.2, -12.0127)
  line L6 (-9, 27.1271) -> (0, 27.1271)
  line L7 (0, 40.3549) -> (0, 0) projected
  circle A1 centre (-3, 32.901) radius 3
  line L8 (-8.7, 22.5305) -> (-8.7, 18.5305) projected
  line L9 (-5.7, 22.5305) -> (-5.7, 18.5305) projected
  line L10 (-9.2, 20.9848) -> (0, 20.9848)
  circle A2 centre (-3, 19.9848) radius 3
  line L11 (-8.7, -0.4409) -> (-8.7, -4.4409) projected
  line L12 (-5.7, -0.4409) -> (-5.7, -4.4409) projected
  line L13 (-9.2, 40.3549) -> (-9.2, -24.9409) projected
  line L14 (-9.2, -0.7765) -> (-2.1, -0.7765)
  line L15 (-2.1, 0) -> (-2.1, -1.8712) projected
  line L16 (-5.5, -20.2285) -> (-5.5, -16.2127) projected
  point P0 (-6.1, -15.7765)
  point P1 (-6.1, -5.7765)
  point P2 (-5.65, -12.0127)
  point P3 (-3.9, 22.6271)
  point P4 (-9, 22.6271)
  point P5 (-8.7, 24.9848)
  point P6 (-8.7, 20.9848)
  point P7 (-5.2, 24.9848)
  point P8 (-5.2, 20.9848)
  point P9 (-8.5, -0.7765)
  point P10 (-8.5, -4.7765)
  point P11 (-6.6, -0.7765)
  point P12 (-6.6, -4.7765)
  point P13 (-9.2, -6.9409)
  point P14 (-5.2, 1.9975)
  point P15 (-5.2, -2.0025)
  point P16 (-6.1, 40.0194)
  point P17 (-6.1, -25.2765)
  point P18 (-2.6, -1.801)
  point P19 (-2.6, -6.7398)
  point P20 (-5.2, 24.9848)
  point P21 (-5.2, 20.9848)
  dimension "d103" = 5.0143
  dimension "d104" = 4.2
  dimension "d105" = 3.55
  dimension "d106" = 3.55
  dimension "d107" = 6
  dimension "d109" = -6.2
  dimension "d110" = 6
  dimension "d113" = 1
  constraints: 8 end point, 6 point on line, 4 horizontal, 2 centre point, 2 tangent, 1 midpoint, 1 perpendicular, 9 other
  measures "d104" distance between parallel lines of L5 L3
  measures "d106" distance from line of L2 point (-5.65, -12.013)
  measures "d107" diameter of A1
  measures "d110" diameter of A2
  measures "d113" distance from line of A2.centre L10
hole "Hole5" at (-23.6, 12.9282, -3.55) at (-23.6, 44.9257, -0.9) at (-23.6, 57.8419, -0.9) at (-23.6, 2.5072, -4.5928) direction (1, 0, 0) diameter 4 depth 3.5 counterbore diameter 4.5 counterbore depth 0.5
sketch "Sketch13" plane through (0, 0, 2.1) normal (1, 0, 0) x (0, 0, -1)
  arc A0 (0, 34.1044) -> (0, 29.1435) centre (-2.1, 31.624) ccw projected
  line L0 (0, 34.1044) -> (0, 35.6915) projected
  arc A1 (0, 40.6523) -> (0, 35.6915) centre (-2.1, 38.1719) ccw projected
  line L1 (0, 40.6523) -> (0, 47.4458) projected
  line L2 (0, 47.4458) -> (-35.3, 47.4458) projected
  line L3 (-35.3, 47.4458) -> (-35.3, 40.6523) projected
  arc A2 (-35.3, 35.6915) -> (-35.3, 40.6523) centre (-33.2, 38.1719) ccw projected
  line L4 (-35.3, 35.6915) -> (-35.3, 34.1044) projected
  arc A3 (-35.3, 29.1435) -> (-35.3, 34.1044) centre (-33.2, 31.624) ccw projected
  line L5 (-35.3, 29.1435) -> (-35.3, 22.35) projected
  line L6 (-35.3, 22.35) -> (0, 22.35) projected
  line L7 (0, 22.35) -> (0, 29.1435) projected
  point P0 (2.1, 0)
hole "Hole6" at (0, 31.624, 4.2) at (0, 38.1719, 4.2) direction (-1, 0, 0) diameter 3.4 depth 8.8 countersink diameter 7 countersink angle 90 clearance for "Countersunk Flat Head Screw ISO 2009/7046" size "M3" standard "ISO"
body "Solid3"
